Autodesk Fusion 360 part; units mm, degrees
(part 6 of 6)
equation "d5795 = b_Tool_diameter"
equation "d5796 = b_Tool_diameter"
equation "d5797 = b_Tool_diameter"
equation "d5798 = b_Tool_diameter"
equation "d5799 = b_Tool_diameter"
equation "d5800 = b_Tool_diameter"
equation "d5802 = b_Thickness"
equation "d5804 = b_Thickness"
equation "d5806 = b_Thickness"
equation "d5808 = b_Thickness"
equation "d5810 = b_Tool_diameter"
equation "d5811 = b_Tool_diameter"
equation "d5812 = b_Tool_diameter"
equation "d5813 = b_Tool_diameter"
equation "d5819 = b_Thickness"
equation "d5821 = b_Thickness"
equation "d5823 = b_Thickness"
equation "d5825 = b_Thickness"
equation "d5827 = b_Thickness"
equation "d5829 = b_Thickness"
equation "d5831 = b_Thickness"
equation "d5833 = b_Thickness"
equation "d5835 = b_Thickness"
equation "d5837 = b_Thickness"
equation "d5839 = b_Tool_diameter"
equation "d5840 = b_Tool_diameter"
equation "d5841 = b_Tool_diameter"
equation "d5842 = b_Tool_diameter"
equation "d5843 = b_Tool_diameter"
equation "d5844 = b_Tool_diameter"
equation "d5845 = b_Tool_diameter"
equation "d5846 = b_Tool_diameter"
equation "d5847 = b_Tool_diameter"
equation "d5848 = b_Tool_diameter"
equation "d5850 = b_Thickness"
equation "d5852 = b_Thickness"
equation "d5854 = b_Thickness"
equation "d5856 = b_Thickness"
equation "d5858 = b_Tool_diameter"
equation "d5859 = b_Tool_diameter"
equation "d5860 = b_Tool_diameter"
equation "d5861 = b_Tool_diameter"
equation "d5863 = b_Thickness"
equation "d5865 = b_Thickness"
equation "d5867 = b_Thickness"
equation "d5869 = b_Thickness"
equation "d5871 = b_Thickness"
equation "d5873 = b_Thickness"
equation "d5875 = b_Thickness"
equation "d5877 = b_Thickness"
equation "d5879 = b_Thickness"
equation "d5881 = b_Thickness"
equation "d5883 = b_Tool_diameter"
equation "d5884 = b_Tool_diameter"
equation "d5885 = b_Tool_diameter"
equation "d5886 = b_Tool_diameter"
equation "d5887 = b_Tool_diameter"
equation "d5888 = b_Tool_diameter"
equation "d5889 = b_Tool_diameter"
equation "d5890 = b_Tool_diameter"
equation "d5891 = b_Tool_diameter"
equation "d5892 = b_Tool_diameter"
equation "d5894 = b_Thickness"
equation "d5896 = b_Thickness"
equation "d5898 = b_Thickness"
equation "d5900 = b_Thickness"
equation "d5902 = b_Tool_diameter"
equation "d5903 = b_Tool_diameter"
equation "d5904 = b_Tool_diameter"
equation "d5905 = b_Tool_diameter"
equation "d5912 = b_Tool_diameter"
equation "d5913 = b_Tool_diameter"
equation "d5917 = ballBearingCenterToCenterVert"
equation "d5918 = ballBearingCenterToCenterHoriz"
equation "d5919 = shaftCenterToCenter"
equation "shaftCenterToCenter = 34 mm"
equation "shaftCenterToMountingHoles = 15.5 mm"
equation "ballBearingHoleDiam = 12.8 mm"
equation "ballBearingCenterToCenterHoriz = 55 mm"
equation "ballBearingCenterToCenterVert = 40 mm"
equation "d5931 = ballBearingHoleDiam"
equation "d5932 = platformMountHoles"
equation "d5933 = shaftCenterToMountingHoles"
equation "d5934 = shaftCenterToMountingHoles"
equation "d5935 = ballBearingHoleDiam"
equation "d5936 = ballBearingCenterToCenterVert"
equation "d5937 = ballBearingCenterToCenterHoriz"
equation "d5938 = shaftCenterToCenter"
equation "d5943 = b_Tool_diameter"
equation "d5959 = platformMountHoles"
equation "d5960 = ( -shaftCenterToCenter + ballBearingCenterToCenterVert ) / 2"
equation "d5967 = platformMountHoles"
equation "d5968 = platformMountHoles"
equation "d5969 = platformMountHoles"
equation "d5970 = platformMountHoles"
equation "d5971 = b_Thickness"
equation "d5973 = pcbMountHoles"
equation "d5974 = 4 mm + b_Thickness"
equation "d5977 = Dlc32Length"
equation "d5979 = Dlc32Length / 2"
equation "d5980 = b_Depth + b_Height + 2 * b_Tool_diameter"
equation "d5981 = b_Depth + b_Tool_diameter"
equation "Dlc32Length = 82 mm"
equation "d5995 = ( b_Length - Dlc32Length ) / 2"
named bodies: "b  stock body", "b top  body", "b top circles cheese body", "b bottom  body", "b bottom circles cheese body", "b front  body", "b front circles cheese body", "b back  body", "b back circles cheese body", "b left  body", "b left circles cheese body", "b right  body", "b right circles cheese body", "platform Body"
